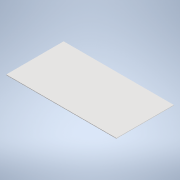
# Autodesk Inventor part: Pieza23
Saved by Autodesk Inventor 2022.2 (Build 262287000, 287)
## iProperties
Created: 2022-02-09
Part Number: Pieza23
Material: Genérico
Document SubType Name: Modeling
Designer: USUARIO
Density: 1 g/cm^3
Appearance: Valor por defecto
Author: USUARIO
Autodesk Inventor part; units mm, degrees
ref_plane "YZ Plane" through (0, 0, 0) normal (1, 0, 0) x (0, 1, 0)
ref_plane "XZ Plane" through (0, 0, 0) normal (0, 1, 0) x (-1, 0, 0)
ref_plane "XY Plane" through (0, 0, 0) normal (0, 0, 1) x (1, 0, 0)
sketch "Boceto1" plane through (0, 0, 0) normal (0, 1, 0) x (-1, 0, 0)
  line L0 (656.793, -1158.0565) -> (58.058, -1158.0565)
  line L1 (58.058, -1158.0565) -> (58.058, -1470.2625)
  line L2 (58.058, -1470.2625) -> (656.793, -1470.2625)
  line L3 (656.793, -1470.2625) -> (656.793, -1158.0565)
  point P0 (0, 0)
  dimension "d0" = 598.735
  dimension "d1" = 312.206
  constraints: 8 end point, 2 parallel, 1 horizontal, 1 perpendicular
  measures "d0" distance of L2.end L1.end
  measures "d1" distance of L1.end L0.end
extrude "Extrusión1" add sketch "Boceto1" along normal blind 3
